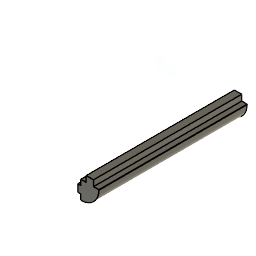
FINAL STOP LIGHT CONNECTOR (Autodesk Fusion 360 design; units mm, degrees)
Autodesk Fusion 360 part; units mm, degrees
sketch "Sketch1" plane through (0, 0, 52.25) normal (0, 0, 1) x (-1, 0, 0)
  line L0 (12.25, -100) -> (12.25, 0)
  line L1 (12.25, 0) -> (0, 0)
  line L2 (0, 0) -> (0, -100)
  line L3 (0, -100) -> (12.25, -100)
  line L4 (0, 0) -> (12.25, 0) construction
  line L5 (6.125, 0) -> (8.625, 0) construction
  line L6 (6.125, 0) -> (3.625, 0) construction
  line L7 (3.625, 0) -> (8.625, 0) construction
  line L8 (3.625, 0) -> (8.625, 0)
  line L9 (8.625, 0) -> (8.625, -100)
  line L10 (8.625, -100) -> (3.625, -100)
  line L11 (3.625, -100) -> (3.625, 0)
  dimension "d3" = 5
  constraint coincident L1.end L2.start
  constraint coincident L0.end L1.start
  constraint midpoint L4 L5.start
  constraint horizontal L8
  constraint vertical L9
  constraint horizontal L10
  constraint vertical L11
  constraint coincident L3 L9.end
  measures "d3" distance of L6.end L5.end
sketch "Sketch2" plane through (0, 100, 0) normal (0, 1, 0) x (-1, 0, 0)
  line L0 (-4, 8.6) -> (-4, 3.6)
  line L1 (-4, 3.6) -> (8.5, 3.6)
  line L2 (8.5, 3.6) -> (8.5, 10.6)
  line L3 (8.5, 10.6) -> (3.5, 10.6)
  line L4 (3.5, 10.6) -> (3.5, 8.6)
  line L5 (3.5, 8.6) -> (-4, 8.6)
sketch "Sketch3" plane through (0, 100, 0) normal (0, 1, 0) x (-1, 0, 0)
  line L0 (-43.625, 52.25) -> (-43.625, 50.25)
  line L1 (-43.625, 50.25) -> (-48.625, 50.25)
  line L2 (-48.625, 50.25) -> (-48.625, 52.25)
  line L3 (-48.625, 52.25) -> (-52.25, 52.25)
  line L4 (-52.25, 52.25) -> (-52.25, 12.25)
  line L5 (-52.25, 12.25) -> (-48.625, 12.25)
  line L6 (-48.625, 12.25) -> (-48.625, 16.25)
  line L7 (-48.625, 16.25) -> (-43.625, 16.25)
  line L8 (-43.625, 16.25) -> (-43.625, 12.25)
  line L9 (-43.625, 12.25) -> (-40, 12.25)
  line L10 (-40, 12.25) -> (-40, 52.25)
  line L11 (-40, 52.25) -> (-43.625, 52.25)
  line L12 (-40, 0) -> (-56, 0) construction
  line L13 (-52.25, 12.25) -> (-48.625, 12.25)
  line L14 (-48.625, 16.25) -> (-48.625, 12.25)
  line L15 (-43.625, 16.25) -> (-48.625, 16.25)
  line L16 (-43.625, 12.25) -> (-43.625, 16.25)
  line L17 (-40, 12.25) -> (-43.625, 12.25)
  line L18 (-40, 8.6) -> (-40, 12.25)
  line L19 (-38, 8.6) -> (-40, 8.6)
  line L20 (-38, 3.6) -> (-38, 8.6)
  line L21 (-40, 3.6) -> (-38, 3.6)
  line L22 (-40, 0) -> (-40, 3.6)
  line L23 (-40, 0) -> (-52.25, 0)
  line L24 (-52.25, 12.25) -> (-52.25, 0)
  constraint coincident L4.end L5.start
  constraint horizontal L12
  constraint coincident L5.end L6.start
  constraint coincident L6.end L7.start
  constraint coincident L7.end L8.start
  constraint coincident L8.end L9.start
  constraint coincident L9.end L10.start
  constraint horizontal L19
  constraint perpendicular L19 L20
  constraint perpendicular L20 L21
  constraint coincident L12 L23.end
extrude "Extrude3" add sketch "Sketch3" against normal blind 100 contours L5 L6 L7 L8 L9 L13 L14 L15 L16 L17 L18 L19 L20 L21 L22 L23 L24
fillet "Fillet1" radius 12 1 edges at (52.25, 50, 0)
